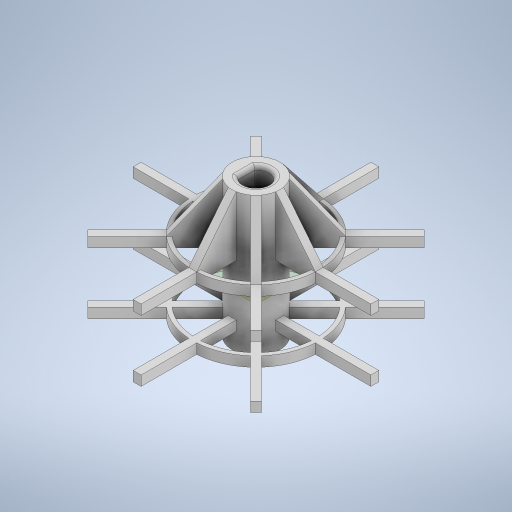
# Autodesk Inventor part: DiseñoRueda_V003
Saved by Autodesk Inventor 2023 (Build 270158000, 158)
## iProperties
Created: 2022-04-27
Part Number: DiseñoRueda_V003
Material: Genérico
Document SubType Name: Modeling
Designer: skatl
Density: 1 g/cm^3
Appearance: Valor por defecto
Author: skatl
Autodesk Inventor part; units mm, degrees
ref_plane "YZ Plane" through (0, 0, 0) normal (1, 0, 0) x (0, 1, 0)
ref_plane "XZ Plane" through (0, 0, 0) normal (0, 1, 0) x (-1, 0, 0)
ref_plane "XY Plane" through (0, 0, 0) normal (0, 0, 1) x (1, 0, 0)
sketch "Boceto1" plane through (0, 0, 0) normal (0, 1, 0) x (-1, 0, 0)
  circle A0 centre (0, 0) radius 3.2
  circle A1 centre (0, 0) radius 6
  line L0 (-3.2, 0) -> (2.4, 0)
  line L1 (2.4, -2.1166) -> (2.4, 2.1166)
  line L2 (2.4, 0) -> (2.4, -2.1166)
  line L3 (3.2, 0) -> (3.2, 1)
  circle A2 centre (0, 0) radius 30
  line L4 (3.2, 1) -> (29.9833, 1)
  line L5 (3.2, 0) -> (3.2, -1)
  line L6 (3.2, -1) -> (29.9833, -1)
  line L7 (1.5556, 2.9698) -> (20.4943, 21.9085)
  line L8 (2.9698, 1.5556) -> (21.9085, 20.4943)
  line L9 (2.2627, 2.2627) -> (1.5556, 2.9698)
  line L10 (2.2627, 2.2627) -> (2.9698, 1.5556)
  line L11 (-1, 3.2) -> (-1, 29.9833)
  line L12 (1, 3.2) -> (1, 29.9833)
  line L13 (0, 3.2) -> (-1, 3.2)
  line L14 (0, 3.2) -> (1, 3.2)
  line L15 (-2.9698, 1.5556) -> (-21.9085, 20.4943)
  line L16 (-1.5556, 2.9698) -> (-20.4943, 21.9085)
  line L17 (-2.2627, 2.2627) -> (-2.9698, 1.5556)
  line L18 (-2.2627, 2.2627) -> (-1.5556, 2.9698)
  line L19 (-3.2, -1) -> (-29.9833, -1)
  line L20 (-3.2, 1) -> (-29.9833, 1)
  line L21 (-3.2, 0) -> (-3.2, -1)
  line L22 (-3.2, 0) -> (-3.2, 1)
  line L23 (-1.5556, -2.9698) -> (-20.4943, -21.9085)
  line L24 (-2.9698, -1.5556) -> (-21.9085, -20.4943)
  line L25 (-2.2627, -2.2627) -> (-1.5556, -2.9698)
  line L26 (-2.2627, -2.2627) -> (-2.9698, -1.5556)
  line L27 (1, -3.2) -> (1, -29.9833)
  line L28 (-1, -3.2) -> (-1, -29.9833)
  line L29 (0, -3.2) -> (1, -3.2)
  line L30 (0, -3.2) -> (-1, -3.2)
  line L31 (2.9698, -1.5556) -> (21.9085, -20.4943)
  line L32 (1.5556, -2.9698) -> (20.4943, -21.9085)
  line L33 (2.2627, -2.2627) -> (2.9698, -1.5556)
  line L34 (2.2627, -2.2627) -> (1.5556, -2.9698)
  circle A3 centre (0, 0) radius 15
  circle A4 centre (0, 0) radius 16
  point P0 (2.4, 0)
  point P1 (3.4762, 4.8904)
  point P2 (1, 5.9161)
  point P3 (1, 29.9833)
  point P4 (-1, 29.9833)
  point P5 (-1, 5.9161)
  point P6 (-3.4762, 4.8904)
  point P7 (-4.8904, 3.4762)
  point P8 (-5.9161, 1)
  point P9 (-29.9833, 1)
  point P10 (-29.9833, -1)
  point P11 (-5.9161, -1)
  point P12 (-4.8904, -3.4762)
  point P13 (-3.4762, -4.8904)
  point P14 (-1, -5.9161)
  point P15 (-1, -29.9833)
  point P16 (1, -29.9833)
  point P17 (1, -5.9161)
  point P18 (3.4762, -4.8904)
  point P19 (4.8904, -3.4762)
  point P20 (5.9161, -1)
  point P21 (29.9833, -1)
  point P22 (5.9161, 1)
  point P23 (4.8904, 3.4762)
  point P24 (11.9987, -10.5845)
  point P25 (15.9687, -1)
  point P26 (14.9666, -1)
  point P27 (11.2901, -9.8759)
  point P28 (1, -15.9687)
  point P29 (10.5845, -11.9987)
  point P30 (9.8759, -11.2901)
  point P31 (1, -14.9666)
  point P32 (-10.5845, -11.9987)
  point P33 (-1, -15.9687)
  point P34 (-1, -14.9666)
  point P35 (-9.8759, -11.2901)
  point P36 (-15.9687, -1)
  point P37 (-11.9987, -10.5845)
  point P38 (-11.2901, -9.8759)
  point P39 (-14.9666, -1)
  point P40 (-11.9987, 10.5845)
  point P41 (-15.9687, 1)
  point P42 (-14.9666, 1)
  point P43 (-11.2901, 9.8759)
  point P44 (-1, 15.9687)
  point P45 (-10.5845, 11.9987)
  point P46 (-9.8759, 11.2901)
  point P47 (-1, 14.9666)
  point P48 (15.9687, 1)
  point P49 (11.9987, 10.5845)
  point P50 (11.2901, 9.8759)
  point P51 (14.9666, 1)
  point P52 (10.5845, 11.9987)
  point P53 (1, 15.9687)
  point P54 (1, 14.9666)
  point P55 (9.8759, 11.2901)
  dimension "d7" = 60
  dimension "d0" = 6.4
  dimension "d1" = 12
  dimension "d2" = 5.6
  dimension "d6" = 1
  dimension "d10" = 360
  dimension "d12" = 30
  dimension "d13" = 32
  constraints: 70 end point, 5 coincident, 4 centre point, 4 point on circle, 2 perpendicular, 2 symmetric about line, 1 horizontal, 1 tangent, 1 vertical, 76 other
  measures "d0" diameter of A0
  measures "d1" diameter of A1
  measures "d2" distance of L0.start L0.end
  measures "d6" distance of L3.start L3.end
  measures "d12" diameter of A3
  measures "d13" diameter of A4
extrude "Extrusión1" add sketch "Boceto1" along normal blind 2.5 contours A0 L1 | L5 L6 A1 L31 L33 A0 | A0 L10 L8 A1 L4 L3 | L3 L4 A1 L6 L5 | A0 L14 L12 A1 L7 L9 | L9 L7 A1 L8 L10 | L34 L32 A1 L27 L29 A0 | L33 L31 A1 L32 L34 | L4 A3 L6 A1 | A0 L18 L16 A1 L11 L13 | L13 L11 A1 L12 L14 | L22 L20 A1 L15 L17 A0 | A0 L26 L24 A1 L19 L21 | L21 L19 A1 L20 L22 | L30 L28 A1 L23 L25 A0 | L29 L27 A1 L28 L30 | A1 L7 A3 L8 | A3 L8 A4 L4 | L4 A4 L6 A3 | L31 A3 L32 A1 | L6 A4 L31 A3 | L17 L15 A1 L16 L18 | L25 L23 A1 L24 L26 | A3 L7 A4 L8 | L4 A2 L6 A4 | L31 A4 L32 A3 | L11 A3 L12 A1 | A3 L12 A4 L7 | L19 A3 L20 A1 | L27 A3 L28 A1 | L32 A4 L27 A3 | A4 L7 A2 L8 | L31 A2 L32 A4 | L15 A3 L16 A1 | A3 L16 A4 L11 | L11 A4 L12 A3 | L23 A3 L24 A1 | A3 L24 A4 L19 | L19 A4 L20 A3 | L20 A4 L15 A3 | L27 A4 L28 A3 | L28 A4 L23 A3 | L15 A4 L16 A3 | L11 A2 L12 A4 | L23 A4 L24 A3 | L19 A2 L20 A4 | L27 A2 L28 A4 | L15 A2 L16 A4 | L23 A2 L24 A4
sketch "Boceto2" plane through (0, 0, 0) normal (0, -1, 0) x (1, 0, 0)
  circle A0 centre (0, 0) radius 3.2
  circle A1 centre (0, 0) radius 6
  line L0 (-3.2, 0) -> (2.4, 0)
  line L1 (2.4, -2.1166) -> (2.4, 2.1166)
  line L2 (2.4, 0) -> (2.4, -2.1166)
  line L3 (3.2, 0) -> (3.2, 1)
  circle A2 centre (0, 0) radius 30
  line L4 (3.2, 1) -> (29.9833, 1)
  line L5 (3.2, -1) -> (29.9833, -1)
  line L6 (3.2, 0) -> (3.2, -1)
  line L7 (1.5556, 2.9698) -> (20.4943, 21.9085)
  line L8 (2.9698, 1.5556) -> (21.9085, 20.4943)
  line L9 (2.2627, 2.2627) -> (1.5556, 2.9698)
  line L10 (2.2627, 2.2627) -> (2.9698, 1.5556)
  line L11 (-1, 3.2) -> (-1, 29.9833)
  line L12 (1, 3.2) -> (1, 29.9833)
  line L13 (0, 3.2) -> (-1, 3.2)
  line L14 (0, 3.2) -> (1, 3.2)
  line L15 (-2.9698, 1.5556) -> (-21.9085, 20.4943)
  line L16 (-1.5556, 2.9698) -> (-20.4943, 21.9085)
  line L17 (-2.2627, 2.2627) -> (-2.9698, 1.5556)
  line L18 (-2.2627, 2.2627) -> (-1.5556, 2.9698)
  line L19 (-3.2, -1) -> (-29.9833, -1)
  line L20 (-3.2, 1) -> (-29.9833, 1)
  line L21 (-3.2, 0) -> (-3.2, -1)
  line L22 (-3.2, 0) -> (-3.2, 1)
  line L23 (-1.5556, -2.9698) -> (-20.4943, -21.9085)
  line L24 (-2.9698, -1.5556) -> (-21.9085, -20.4943)
  line L25 (-2.2627, -2.2627) -> (-1.5556, -2.9698)
  line L26 (-2.2627, -2.2627) -> (-2.9698, -1.5556)
  line L27 (1, -3.2) -> (1, -29.9833)
  line L28 (-1, -3.2) -> (-1, -29.9833)
  line L29 (0, -3.2) -> (1, -3.2)
  line L30 (0, -3.2) -> (-1, -3.2)
  line L31 (2.9698, -1.5556) -> (21.9085, -20.4943)
  line L32 (1.5556, -2.9698) -> (20.4943, -21.9085)
  line L33 (2.2627, -2.2627) -> (2.9698, -1.5556)
  line L34 (2.2627, -2.2627) -> (1.5556, -2.9698)
  circle A3 centre (0, 0) radius 15
  circle A4 centre (0, 0) radius 16
  line L35 (0, 0) -> (0, 2.0135)
  line L36 (-2.4, -2.1166) -> (-2.4, 2.1166)
  point P0 (-2.4, -2.1166)
  point P1 (-2.4, 2.1166)
  dimension "d20" = 60
  dimension "d16" = 6.4
  dimension "d17" = 12
  dimension "d18" = 5.6
  dimension "d19" = 1
  dimension "d21" = 360
  dimension "d22" = 30
  dimension "d23" = 32
  constraints: 74 end point, 5 coincident, 4 centre point, 4 point on circle, 4 symmetric about line, 2 perpendicular, 2 vertical, 1 horizontal, 1 tangent, 76 other
  measures "d16" diameter of A0
  measures "d17" diameter of A1
  measures "d18" distance of L0.start L0.end
  measures "d19" distance of L6.start L3.end
  measures "d22" diameter of A3
  measures "d23" diameter of A4
extrude "Extrusión2" add sketch "Boceto2" along normal blind 20 and the other way blind 15 contours L6 L5 A1 L31 L33 A0 | A0 L10 L8 A1 L4 L3 | L3 L4 A1 L5 L6 | A0 L14 L12 A1 L7 L9 | L9 L7 A1 L8 L10 | L34 L32 A1 L27 L29 A0 | L33 L31 A1 L32 L34 | A0 L18 L16 A1 L11 L13 | L13 L11 A1 L12 L14 | L30 L28 A1 L23 L25 A0 | L29 L27 A1 L28 L30 | A0 L22 L20 A1 L15 L17 | L17 L15 A1 L16 L18 | L36 A0 L0 | L0 A0 L36 | L26 L24 A1 L19 L21 A0 | L25 L23 A1 L24 L26 | L21 L19 A1 L20 L22
ref_plane "Plano de trabajo1" through (0, -6.5, 0) normal (0, -1, 0) x (1, 0, 0)
mirror "Simetría1" about plane through (0, -6.5, 0) normal (0, -1, 0) of "Extrusión1"
sketch "Boceto5" plane through (0, 0, 0) normal (1, 0, 0) x (0, 1, 0)
  line L0 (-20, 6) -> (15, 6) projected
  line L1 (0, 15.9687) -> (2.5, 15.9687) projected
  line L2 (15, 6) -> (2.5, 15.9687)
  line L3 (2.5, 15.9687) -> (2.5, 6)
  line L4 (2.5, 6) -> (15, 6)
  line L5 (15, 6) -> (15, 5.2503)
  line L6 (15, 5.2503) -> (2.5, 5.2503)
  line L7 (2.5, 1) -> (2.5, 10.5845) projected
  point P0 (0, 0)
  constraints: 10 end point, 2 perpendicular, 2 point on line, 2 vertical
extrude "Extrusión5" add sketch "Boceto5" along normal mid plane 2
pattern_circular "Patrón circular1" count 6 over 225 about axis through (0, -10, 0) along (0, 1, 0) of "Extrusión5"
pattern_circular "Patrón circular2" count 2 over 45 about axis through (0, -10, 0) along (0, -1, 0) of "Extrusión5"
sketch "Boceto6" plane through (-2.4, -20, -2.1166) normal (1, 0, 0) x (0, 0, -1)
  line L0 (-4.2332, 35) -> (0, 35) projected
  line L1 (-2.1166, 35) -> (-2.1166, 22.5)
  line L2 (-3.1166, 22.5) -> (-1.1166, 22.5) projected
  line L3 (-2.1166, 35) -> (-2.1166, 30)
  circle A0 centre (-2.1166, 30) radius 1.35
  point P0 (-2.1166, 20)
  dimension "d54" = 5
  dimension "d55" = 2.7
  constraints: 4 end point, 2 midpoint, 1 centre point, 1 coincident, 1 point on line
  measures "d54" distance of L1.start L3.end
  measures "d55" diameter of A0
extrude "Extrusión6" cut sketch "Boceto6" against normal through all
fillet "Empalme2" radius 1 2 edges at (3.2, 15, 0) (-2.4, 15, 0)
fillet "Empalme3" radius 1 2 edges at (3.2, -20, 0) (-2.4, -20, 0)
